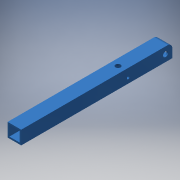
# Autodesk Inventor part: pivot arm
Saved by Autodesk Inventor 2017 SP1 (Build 210196100, 196)
## iProperties
Created: 2018-01-25
Part Number: pivot arm
Material: Aluminum 6061
Document SubType Name: Modeling
Designer: Ben
Density: 2.7 g/cm^3
Appearance: Cyan
Mass: 210.518 g
Surface Area: 502.922 cm^2
Volume: 77.9696 cm^3
Author: Ben
Autodesk Inventor part; units mm, degrees
ref_plane "YZ Plane" through (0, 0, 0) normal (1, 0, 0) x (0, 1, 0)
ref_plane "XZ Plane" through (0, 0, 0) normal (0, 1, 0) x (-1, 0, 0)
ref_plane "XY Plane" through (0, 0, 0) normal (0, 0, 1) x (1, 0, 0)
sketch "Sketch1" plane through (0, 0, 0) normal (0, 0, 1) x (1, 0, 0)
  line L0 (-12.7, -12.7) -> (12.7, -12.7)
  line L1 (12.7, -12.7) -> (12.7, 12.7)
  line L2 (12.7, 12.7) -> (-12.7, 12.7)
  line L3 (-12.7, 12.7) -> (-12.7, -12.7)
  line L4 (-12.7, -12.7) -> (12.7, 12.7) construction
  line L5 (12.7, -12.7) -> (-12.7, 12.7) construction
  line L6 (-9.525, -9.525) -> (9.525, -9.525)
  line L7 (9.525, -9.525) -> (9.525, 9.525)
  line L8 (9.525, 9.525) -> (-9.525, 9.525)
  line L9 (-9.525, 9.525) -> (-9.525, -9.525)
  line L10 (-9.525, -9.525) -> (9.525, 9.525) construction
  line L11 (9.525, -9.525) -> (-9.525, 9.525) construction
  point P0 (0, 0)
  dimension "d0" = 25.4
  dimension "d1" = 3.175
  constraints: 24 end point, 4 midpoint, 4 parallel, 3 perpendicular, 2 horizontal, 1 point on line
  measures "d0" distance of L0.end L1.end
  measures "d1" distance between parallel lines of L1 L7
extrude "Extrusion1" add sketch "Sketch1" along normal mid plane 282.575
sketch "Sketch2" plane through (12.7, -12.7, 141.2875) normal (1, 0, 0) x (0, 0, -1)
  line L0 (0, 22.225) -> (0, 3.175) construction
  line L1 (0, 12.7) -> (282.575, 12.7) construction
  line L2 (282.575, 3.175) -> (282.575, 22.225) construction
  circle A0 centre (269.875, 12.7) radius 4.7625
  circle A1 centre (200.025, 9.525) radius 2.54
  point P0 (141.2875, 12.7)
  dimension "d4" = 9.525
  dimension "d5" = 12.7
  dimension "d19" = 5.08
  dimension "d20" = 69.85
  dimension "d21" = 3.175
  constraints: 2 centre point, 2 end point, 2 midpoint, 1 point on line
  measures "d4" diameter of A0
  measures "d5" distance from line of L2 A0.centre
  measures "d19" diameter of A1
  measures "d20" horizontal distance of A0.centre A1.centre
  measures "d21" distance from line of A1.centre L1
extrude "Extrusion2" cut sketch "Sketch2" against normal through all
sketch "Sketch3" plane through (-12.7, 12.7, 141.2875) normal (0, 1, 0) x (1, 0, 0)
  line L0 (0, 0) -> (25.4, 0) construction
  line L1 (22.225, 282.575) -> (3.175, 282.575) construction
  line L2 (0, 282.575) -> (0, 0) projected
  line L3 (3.175, 282.575) -> (22.225, 282.575) construction
  line L4 (3.175, 282.575) -> (3.175, 0) construction
  circle A0 centre (12.7, 193.675) radius 4.7625
  line L5 (25.4, 282.575) -> (25.4, 0) projected
  point P0 (12.7, 141.2875)
  dimension "d15" = 3.175
  dimension "d22" = 88.9
  dimension "d23" = 12.7
  dimension "d24" = 9.525
  constraints: 2 end point, 2 point on line, 1 centre point, 1 vertical
  measures "d15" distance between parallel lines of L2 L4
  measures "d22" distance from line of L1 A0.centre
  measures "d23" distance from line of L2 A0.centre
  measures "d24" diameter of A0
extrude "Extrusion3" cut sketch "Sketch3" against normal through all
fillet "Fillet1" radius 9.525 1 edges at (0, 12.7, -141.2875)
body "Solid1"
